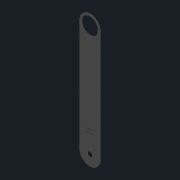
# Autodesk Inventor part: link2-plate1
Saved by Autodesk Inventor 2021 (Build 250183000, 183)
## iProperties
Created: 2021-07-15
Part Number: link2-plate1
Material: CFRP
Document SubType Name: Sheet Metal
Designer: yuta0
Density: 1.43 g/cm^3
Sheet Metal Rule: Default
Appearance: カーボンファイバー
Mass: 107.591 g
Surface Area: 786.154 cm^2
Volume: 75.2383 cm^3
Author: yuta0
Autodesk Inventor part; units mm, degrees
ref_plane "YZ Plane" through (0, 0, 0) normal (1, 0, 0) x (0, 1, 0)
ref_plane "XZ Plane" through (0, 0, 0) normal (0, 1, 0) x (-1, 0, 0)
ref_plane "XY Plane" through (0, 0, 0) normal (0, 0, 1) x (1, 0, 0)
sketch "スケッチ1" plane through (0, 0, 0) normal (0, 0, 1) x (1, 0, 0)
  circle A0 centre (0, 0) radius 40.5
  circle A1 centre (0, 440) radius 40.5
  line L0 (-40.5, 0) -> (-40.5, 440)
  line L1 (40.5, 440) -> (40.5, 0)
  dimension "d0" = 81
  dimension "d1" = 81
  dimension "d2" = 440
  measures "d0" diameter of A0
  measures "d1" diameter of A1
  measures "d2" distance of A0.centre A1.centre
extrude "プレート1" add sketch "スケッチ1" along normal blind 2
sketch "スケッチ6" plane through (0, 0, 2) normal (0, 0, 1) x (1, 0, 0)
  arc A0 (40.5, 440) -> (-40.5, 440) centre (0, 440) ccw projected
  circle A1 centre (0, 440) radius 32.5
  point P0 (0, 0)
  dimension "d43" = 65
  constraints: 1 centre point, 1 coincident
  measures "d43" diameter of A1
extrude "押し出し2" cut sketch "スケッチ6" against normal blind 10
sketch "スケッチ7" plane through (0, 0, 2) normal (0, 0, 1) x (1, 0, 0)
  arc A0 (40.5, 440) -> (-40.5, 440) centre (0, 440) ccw projected
  circle A1 centre (0, 440) radius 36.5
  point P0 (0, 0)
  point P1 (0, 476.5)
  point P2 (-31.6099, 458.25)
  point P3 (-31.6099, 421.75)
  point P4 (0, 403.5)
  point P5 (31.6099, 421.75)
  point P6 (31.6099, 458.25)
  dimension "d46" = 73
  dimension "d49" = 360
  constraints: 1 coincident, 1 vertical alignment, 9 other
hole "穴4" at (0, 476.5, 2) at (-31.6099, 458.25, 2) at (-31.6099, 421.75, 2) at (0, 403.5, 2) at (31.6099, 421.75, 2) at (31.6099, 458.25, 2) direction (0, 0, -1) diameter 3.2 end through all clearance for "Socket Head Cap Screw" size "M3" standard "Ansi Metric M Profile"
sketch "スケッチ8" plane through (0, 0, 2) normal (0, 0, 1) x (1, 0, 0)
  arc A0 (40.5, 440) -> (-40.5, 440) centre (0, 440) ccw projected
  circle A1 centre (0, 440) radius 25
  line L0 (23.4923, 431.4495) -> (-32.7335, 276.9703)
  line L1 (-23.4923, 448.5505) -> (-36.9957, 411.4503)
  line L2 (0, 603.9) -> (0, -147.9) projected
  circle A2 centre (0, 355.2097) radius 4
  point P0 (0, 0)
  point P1 (4, 72)
  dimension "d92" = 50
  dimension "d93" = 20
  dimension "d94" = 8
  dimension "d102" = 0
  dimension "d140" = 72
  dimension "d141" = 4
  constraints: 4 end point, 3 tangent, 2 centre point, 2 coincident, 2 point on circle, 1 parallel
  measures "d92" diameter of A1
  measures "d93" angle of L2 L0
  measures "d94" diameter of A2
  measures "d102" distance from line of L2 A2.centre
  measures "d140" vertical distance of point (0, 0) point (4, 72)
  measures "d141" horizontal distance of point (0, 0) point (4, 72)
hole "穴5" at (4, 72, 2) at (0, 355.2097, 2) direction (0, 0, -1) diameter 4.3 end through all clearance for "Socket Head Cap Screw" size "M4" standard "Ansi Metric M Profile"
sketch "スケッチ9" plane through (0, 0, 2) normal (0, 0, 1) x (1, 0, 0)
  circle A0 centre (0, 0) radius 67.5
  circle A1 centre (9, 84) radius 8
  arc A2 (40.5, 440) -> (-40.5, 440) centre (0, 440) ccw projected
  dimension "d69" = 84
  dimension "d79" = 135
  dimension "d80" = 16
  dimension "d144" = 9
  constraints: 2 centre point, 2 coincident
  measures "d69" vertical distance of point (0, 0) point (9, 84)
  measures "d79" diameter of A0
  measures "d80" diameter of A1
  measures "d144" horizontal distance of point (0, 0) point (9, 84)
hole "穴6" at (9, 84, 2) direction (0, 0, -1) diameter 4.3 end through all clearance for "Flat Head Machine Screw" size "M4" standard "Ansi Metric M Profile"
sketch "スケッチ13" plane through (0, 0, 2) normal (0, 0, 1) x (1, 0, 0)
  circle A0 centre (0, 0) radius 15
  point P0 (0, 15)
  point P1 (-12.9904, 7.5)
  point P2 (-12.9904, -7.5)
  point P3 (0, -15)
  point P4 (12.9904, -7.5)
  point P5 (12.9904, 7.5)
  dimension "d109" = 30
  dimension "d112" = 360
  constraints: 1 coincident, 1 vertical alignment, 9 other
hole "穴8" at (0, 15, 2) at (-12.9904, 7.5, 2) at (-12.9904, -7.5, 2) at (0, -15, 2) at (12.9904, -7.5, 2) at (12.9904, 7.5, 2) direction (0, 0, -1) diameter 3.4 end through all clearance for "Flat Head Machine Screw" size "M3" standard "Ansi Metric M Profile"
sketch "スケッチ14" plane through (0, 0, 2) normal (0, 0, 1) x (1, 0, 0)
  circle A0 centre (0, 0) radius 10
  dimension "d121" = 20
  constraints: 1 centre point, 1 coincident
  measures "d121" diameter of A0
extrude "押し出し5" cut sketch "スケッチ14" against normal blind 10
sketch "スケッチ15" plane through (0, 0, 2) normal (0, 0, 1) x (1, 0, 0)
  line L0 (-16, 84) -> (9, 84) construction
  line L1 (-16, 81.85) -> (9, 81.85)
  line L2 (9, 86.15) -> (-16, 86.15)
  arc A0 (-16, 86.15) -> (-16, 81.85) centre (-16, 84) ccw
  arc A1 (9, 81.85) -> (9, 86.15) centre (9, 84) ccw
  circle A2 centre (9, 84) radius 2.15 projected
  point P0 (0, 0)
  dimension "d142" = 25
  constraints: 8 end point, 5 tangent, 4 point on circle, 2 centre point, 1 coincident, 1 horizontal, 1 parallel
  measures "d142" distance of L0.start L0.end
extrude "押し出し6" cut sketch "スケッチ15" against normal blind 10
sketch "スケッチ17" plane through (0, 0, 0) normal (0, 0, -1) x (-1, 0, 0)
  point P0 (0, 0)
  point P1 (0, 220)
  dimension "d132" = 220
  measures "d132" distance of point (0, 0) point (0, 220)
hole "穴9" at (0, 220, 0) direction (0, 0, 1) diameter 4.5 end through all clearance for "Flat Head Machine Screw" size "M4" standard "Ansi Metric M Profile"
sketch "スケッチ16" plane through (0, 0, 2) normal (0, 0, 1) x (1, 0, 0)
  line L0 (-21, 72) -> (4, 72) construction
  line L1 (-21, 69.85) -> (4, 69.85)
  line L2 (4, 74.15) -> (-21, 74.15)
  arc A0 (-21, 74.15) -> (-21, 69.85) centre (-21, 72) ccw
  arc A1 (4, 69.85) -> (4, 74.15) centre (4, 72) ccw
  circle A2 centre (4, 72) radius 2.15 projected
  point P0 (0, 0)
  point P1 (-8.5, 72)
  dimension "d143" = 21
  constraints: 8 end point, 5 tangent, 4 point on circle, 2 centre point, 1 coincident, 1 horizontal, 1 midpoint, 1 parallel
  measures "d143" horizontal distance of L0.start point (0, 0)
extrude "押し出し7" cut sketch "スケッチ16" against normal blind 10
equation "\"d56\" = Thickness"
equation "\"d67\" = Thickness"
equation "\"d77\" = Thickness"
equation "\"d119\" = Thickness"
equation "\"d138\" = Thickness"
equation "\"d3\" = Thickness"
equation "\"BendRadius\" = Thickness"
equation "\"BendReliefWidth\" = Thickness"
equation "\"BendReliefDepth\" = 0.5 * Thickness"
equation "\"CornerReliefSize\" = 4 * Thickness"
equation "\"MinimumRemnant\" = 2 * Thickness"
equation "\"TransitionRadius\" = BendRadius"
equation "\"JacobiRadiusSize\" = Thickness"
equation "\"GapSize\" = Thickness"
equation "\"Thickness\" = 2"
